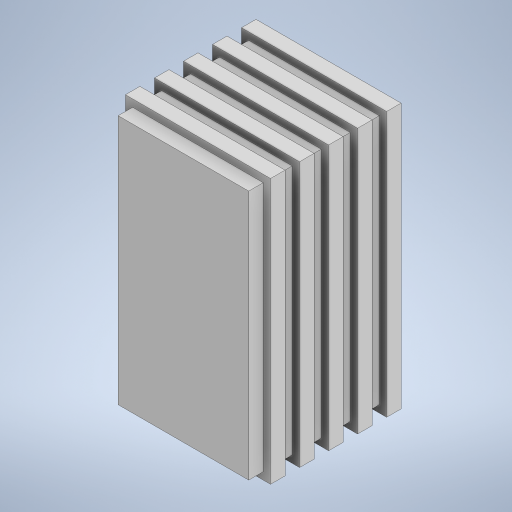
# Autodesk Inventor part: 連接件1
Saved by Autodesk Inventor 2024 (Build 280153000, 153)
## iProperties
Created: 2024-05-23
Part Number: 連接件1
Material: 一般
Document SubType Name: Modeling
Designer: User
Density: 1 g/cm^3
Appearance: 預設
Author: User
Autodesk Inventor part; units mm, degrees
ref_plane "YZ Plane" through (0, 0, 0) normal (1, 0, 0) x (0, 1, 0)
ref_plane "XZ Plane" through (0, 0, 0) normal (0, 1, 0) x (-1, 0, 0)
ref_plane "XY Plane" through (0, 0, 0) normal (0, 0, 1) x (1, 0, 0)
sketch "草圖1" plane through (0, 0, 0) normal (0, 0, 1) x (1, 0, 0)
  line L0 (0, 0) -> (20, 0)
  line L1 (20, 0) -> (20, -36.5)
  line L2 (20, -36.5) -> (0, -36.5)
  line L3 (0, -36.5) -> (0, 0)
  dimension "d0" = 20
  dimension "d1" = 36.5
  constraints: 8 end point, 2 parallel, 1 horizontal, 1 perpendicular
  measures "d0" distance of L1.end L2.end
  measures "d1" distance of L0.end L1.end
extrude "擠出1" add sketch "草圖1" along normal blind 2
sketch "草圖2" plane through (0, 0, 2) normal (0, 0, 1) x (1, 0, 0)
  line L0 (1, -1) -> (19, -1)
  line L1 (19, -1) -> (19, -35.5)
  line L2 (19, -35.5) -> (1, -35.5)
  line L3 (1, -35.5) -> (1, -1)
  line L4 (20, 0) -> (0, 0) projected
  line L5 (20, -36.5) -> (20, 0) projected
  line L6 (0, -36.5) -> (20, -36.5) projected
  line L7 (0, 0) -> (0, -36.5) projected
  dimension "d4" = 1
  dimension "d5" = 1
  dimension "d6" = 1
  dimension "d7" = 1
  constraints: 8 end point, 2 parallel, 1 horizontal, 1 perpendicular
  measures "d4" distance between parallel lines of L4 L0
  measures "d5" distance between parallel lines of L5 L1
  measures "d6" distance between parallel lines of L6 L2
  measures "d7" distance between parallel lines of L7 L3
extrude "擠出2" add sketch "草圖2" along normal blind 2 contours L0 L1 L2 L3
sketch "草圖3" plane through (0, 0, 4) normal (0, 0, 1) x (1, 0, 0)
  line L0 (20, -36.5) -> (20, 0) projected
  line L1 (0, 0) -> (20, 0)
  line L2 (20, 0) -> (20, -36.5)
  line L3 (20, -36.5) -> (0, -36.5)
  line L4 (0, -36.5) -> (0, 0)
  constraints: 8 end point, 2 parallel, 1 horizontal, 1 perpendicular
extrude "擠出3" add sketch "草圖3" along normal blind 2
sketch "草圖4" plane through (0, 0, 6) normal (0, 0, 1) x (1, 0, 0)
  line L0 (1, -35.5) -> (1, -1) projected
  line L1 (19, -1) -> (19, -35.5) projected
  line L2 (1, -1) -> (19, -1)
  line L3 (19, -1) -> (19, -35.5)
  line L4 (19, -35.5) -> (1, -35.5)
  line L5 (1, -35.5) -> (1, -1)
  point P0 (0, 0)
  constraints: 8 end point, 2 parallel, 1 horizontal, 1 perpendicular
extrude "擠出4" add sketch "草圖4" along normal blind 2
sketch "草圖5" plane through (0, 0, 8) normal (0, 0, 1) x (1, 0, 0)
  line L0 (20, -36.5) -> (20, 0) projected
  line L1 (0, 0) -> (20, 0)
  line L2 (20, 0) -> (20, -36.5)
  line L3 (20, -36.5) -> (0, -36.5)
  line L4 (0, -36.5) -> (0, 0)
  constraints: 8 end point, 2 parallel, 1 horizontal, 1 perpendicular
extrude "擠出5" add sketch "草圖5" along normal blind 2
sketch "草圖6" plane through (0, 0, 10) normal (0, 0, 1) x (1, 0, 0)
  line L0 (1, -1) -> (19, -1) projected
  line L1 (19, -35.5) -> (1, -35.5) projected
  line L2 (1, -1) -> (19, -1)
  line L3 (19, -1) -> (19, -35.5)
  line L4 (19, -35.5) -> (1, -35.5)
  line L5 (1, -35.5) -> (1, -1)
  point P0 (0, 0)
  constraints: 8 end point, 2 parallel, 1 horizontal, 1 perpendicular
extrude "擠出6" add sketch "草圖6" along normal blind 2
sketch "草圖7" plane through (0, 0, 0) normal (0, 0, -1) x (-1, 0, 0)
  line L0 (-19, -1) -> (-19, -35.5) projected
  line L1 (-1, -1) -> (-1, -35.5) projected
  line L2 (-19, -1) -> (-1, -1)
  line L3 (-1, -1) -> (-1, -35.5)
  line L4 (-1, -35.5) -> (-19, -35.5)
  line L5 (-19, -35.5) -> (-19, -1)
  point P0 (0, 0)
  constraints: 8 end point, 2 parallel, 1 horizontal, 1 perpendicular
extrude "擠出7" add sketch "草圖7" along normal blind 2
sketch "草圖8" plane through (0, 0, -2) normal (0, 0, -1) x (-1, 0, 0)
  line L0 (0, 0) -> (0, -36.5) projected
  line L1 (-20, 0) -> (0, 0)
  line L2 (0, 0) -> (0, -36.5)
  line L3 (0, -36.5) -> (-20, -36.5)
  line L4 (-20, -36.5) -> (-20, 0)
  constraints: 8 end point, 2 parallel, 1 horizontal, 1 perpendicular
extrude "擠出8" add sketch "草圖8" along normal blind 2
sketch "草圖9" plane through (0, 0, -4) normal (0, 0, -1) x (-1, 0, 0)
  line L0 (-1, -1) -> (-1, -35.5) projected
  line L1 (-19, -1) -> (-1, -1)
  line L2 (-1, -1) -> (-1, -35.5)
  line L3 (-1, -35.5) -> (-19, -35.5)
  line L4 (-19, -35.5) -> (-19, -1)
  point P0 (0, 0)
  constraints: 8 end point, 2 parallel, 1 horizontal, 1 perpendicular
extrude "擠出9" add sketch "草圖9" along normal blind 2
sketch "草圖10" plane through (0, 0, -6) normal (0, 0, -1) x (-1, 0, 0)
  line L0 (0, 0) -> (-20, 0) projected
  line L1 (0, -36.5) -> (0, 0) projected
  line L2 (-20, 0) -> (0, 0)
  line L3 (0, 0) -> (0, -36.5)
  line L4 (0, -36.5) -> (-20, -36.5)
  line L5 (-20, -36.5) -> (-20, 0)
  constraints: 8 end point, 2 parallel, 1 horizontal, 1 perpendicular
extrude "擠出10" add sketch "草圖10" along normal blind 2
